10 pillar (Autodesk Fusion 360 design; units mm, degrees)
description: Spur Gear; Module: 1.27; Num Teeth: 11; Pressure Angle: 20.0; Backlash: 0.00 mm
part number: 2026-06-06-15-54-31-604
Autodesk Fusion 360 part; units mm, degrees
pattern_circular "C-Pattern1" [no effect]
sketch "Base Circle" plane through (0, 0, 0) normal (0, 0, 1) x (1, 0, 0)
  circle A0 centre (0, 0) radius 4.8806
  circle A1 centre (0, 0) radius 2.5
extrude "Extrude4" add sketch "Base Circle" along normal blind 1
sketch "Gear Tooth" plane through (0, 0, 0) normal (0, 0, 1) x (1, 0, 0)
  spline S0 degree 5 poles (5.879, -1.0212) (5.8838, -1.022) (5.8935, -1.0235) (5.908, -1.0253) (5.9275, -1.0267) (5.952, -1.0272) (5.9766, -1.0267) (6.0013, -1.0257) (6.026, -1.0244) (6.0508, -1.0228) (6.0756, -1.021) (6.1004, -1.0189) (6.1253, -1.0165) (6.1502, -1.0135) (6.1752, -1.0101) (6.2001, -1.0063) (6.2251, -1.002) (6.2502, -0.9975) (6.2752, -0.9927) (6.3003, -0.9876) (6.3253, -0.9823) (6.3504, -0.9767) (6.3755, -0.9708) (6.4006, -0.9646) (6.4257, -0.9581) (6.4508, -0.9513) (6.4759, -0.9442) (6.501, -0.9369) (6.5261, -0.9293) (6.5512, -0.9215) (6.5763, -0.9134) (6.6014, -0.9051) (6.6265, -0.8965) (6.6516, -0.8877) (6.6767, -0.8786) (6.7018, -0.8693) (6.7268, -0.8598) (6.7519, -0.85) (6.7769, -0.84) (6.8019, -0.8297) (6.8269, -0.8193) (6.8519, -0.8086) (6.8768, -0.7977) (6.9017, -0.7865) (6.9267, -0.7752) (6.9515, -0.7636) (6.9764, -0.7518) (7.0012, -0.7398) (7.0261, -0.7275) (7.0508, -0.7151) (7.0756, -0.7025) (7.1003, -0.6896) (7.125, -0.6765) (7.1497, -0.6632) (7.1743, -0.6498) (7.1989, -0.6361) (7.2235, -0.6222) (7.248, -0.6081) (7.2725, -0.5938) (7.2969, -0.5793) (7.3213, -0.5646) (7.3457, -0.5497) (7.37, -0.5346) (7.3943, -0.5193) (7.4186, -0.5038) (7.4428, -0.4882) (7.4669, -0.4723) (7.491, -0.4562) (7.5151, -0.44) (7.5391, -0.4236) (7.5631, -0.4069) (7.5822, -0.3935) (7.5966, -0.3833) (7.6061, -0.3765) (7.6109, -0.373) knots 0 0 0 0 0 0 0.01428571 0.02857143 0.04285714 0.05714286 0.07142857 0.08571429 0.1 0.11428571 0.12857143 0.14285714 0.15714286 0.17142857 0.18571429 0.2 0.21428571 0.22857143 0.24285714 0.25714286 0.27142857 0.28571429 0.3 0.31428571 0.32857143 0.34285714 0.35714286 0.37142857 0.38571429 0.4 0.41428571 0.42857143 0.44285714 0.45714286 0.47142857 0.48571429 0.5 0.51428571 0.52857143 0.54285714 0.55714286 0.57142857 0.58571429 0.6 0.61428571 0.62857143 0.64285714 0.65714286 0.67142857 0.68571429 0.7 0.71428571 0.72857143 0.74285714 0.75714286 0.77142857 0.78571429 0.8 0.81428571 0.82857143 0.84285714 0.85714286 0.87142857 0.88571429 0.9 0.91428571 0.92857143 0.94285714 0.95714286 0.97142857 0.98571429 1 1 1 1 1 1
  spline S1 degree 5 poles (5.879, 1.0212) (5.8838, 1.022) (5.8935, 1.0235) (5.908, 1.0253) (5.9275, 1.0267) (5.952, 1.0272) (5.9766, 1.0267) (6.0013, 1.0257) (6.026, 1.0244) (6.0508, 1.0228) (6.0756, 1.021) (6.1004, 1.0189) (6.1253, 1.0165) (6.1502, 1.0135) (6.1752, 1.0101) (6.2001, 1.0063) (6.2251, 1.002) (6.2502, 0.9975) (6.2752, 0.9927) (6.3003, 0.9876) (6.3253, 0.9823) (6.3504, 0.9767) (6.3755, 0.9708) (6.4006, 0.9646) (6.4257, 0.9581) (6.4508, 0.9513) (6.4759, 0.9442) (6.501, 0.9369) (6.5261, 0.9293) (6.5512, 0.9215) (6.5763, 0.9134) (6.6014, 0.9051) (6.6265, 0.8965) (6.6516, 0.8877) (6.6767, 0.8786) (6.7018, 0.8693) (6.7268, 0.8598) (6.7519, 0.85) (6.7769, 0.84) (6.8019, 0.8297) (6.8269, 0.8193) (6.8519, 0.8086) (6.8768, 0.7977) (6.9017, 0.7865) (6.9267, 0.7752) (6.9515, 0.7636) (6.9764, 0.7518) (7.0012, 0.7398) (7.0261, 0.7275) (7.0508, 0.7151) (7.0756, 0.7025) (7.1003, 0.6896) (7.125, 0.6765) (7.1497, 0.6632) (7.1743, 0.6498) (7.1989, 0.6361) (7.2235, 0.6222) (7.248, 0.6081) (7.2725, 0.5938) (7.2969, 0.5793) (7.3213, 0.5646) (7.3457, 0.5497) (7.37, 0.5346) (7.3943, 0.5193) (7.4186, 0.5038) (7.4428, 0.4882) (7.4669, 0.4723) (7.491, 0.4562) (7.5151, 0.44) (7.5391, 0.4236) (7.5631, 0.4069) (7.5822, 0.3935) (7.5966, 0.3833) (7.6061, 0.3765) (7.6109, 0.373) knots 0 0 0 0 0 0 0.01428571 0.02857143 0.04285714 0.05714286 0.07142857 0.08571429 0.1 0.11428571 0.12857143 0.14285714 0.15714286 0.17142857 0.18571429 0.2 0.21428571 0.22857143 0.24285714 0.25714286 0.27142857 0.28571429 0.3 0.31428571 0.32857143 0.34285714 0.35714286 0.37142857 0.38571429 0.4 0.41428571 0.42857143 0.44285714 0.45714286 0.47142857 0.48571429 0.5 0.51428571 0.52857143 0.54285714 0.55714286 0.57142857 0.58571429 0.6 0.61428571 0.62857143 0.64285714 0.65714286 0.67142857 0.68571429 0.7 0.71428571 0.72857143 0.74285714 0.75714286 0.77142857 0.78571429 0.8 0.81428571 0.82857143 0.84285714 0.85714286 0.87142857 0.88571429 0.9 0.91428571 0.92857143 0.94285714 0.95714286 0.97142857 0.98571429 1 1 1 1 1 1
  arc A0 (7.6109, -0.373) -> (7.6109, 0.373) centre (0, 0) ccw
  line L0 (4.7988, -0.8335) -> (5.879, -1.0212)
  line L1 (4.7988, 0.8335) -> (5.879, 1.0212)
  line L2 (4.7988, -0.8335) -> (4.7988, 0.8335)
  point P0 (5.998, -1.0258)
  point P1 (6.1192, -1.017)
  point P2 (6.2418, -0.999)
  point P3 (6.3654, -0.9731)
  point P4 (6.4896, -0.9402)
  point P5 (6.6144, -0.9006)
  point P6 (6.7395, -0.8548)
  point P7 (6.8648, -0.8029)
  point P8 (6.9901, -0.7452)
  point P9 (7.1151, -0.6817)
  point P10 (7.2399, -0.6127)
  point P11 (7.3642, -0.5382)
  point P12 (7.4879, -0.4583)
  point P13 (5.998, 1.0258)
  point P14 (6.1192, 1.017)
  point P15 (6.2418, 0.999)
  point P16 (6.3654, 0.9731)
  point P17 (6.4896, 0.9402)
  point P18 (6.6144, 0.9006)
  point P19 (6.7395, 0.8548)
  point P20 (6.8648, 0.8029)
  point P21 (6.9901, 0.7452)
  point P22 (7.1151, 0.6817)
  point P23 (7.2399, 0.6127)
  point P24 (7.3642, 0.5382)
  point P25 (7.4879, 0.4583)
extrude "Extrude5" add sketch "Gear Tooth" along normal blind 1
fillet "Fillet2" radius 0.2 2 edges at (4.8086, -0.8353, 0.5) (4.8086, 0.8353, 0.5)
pattern_circular "C-Pattern2" count 10 over 360 about axis through (0, 0, 0) along (0, 0, 1) of "Extrude5", "Fillet2"
sketch "Diametrial Pitch Circle" plane through (0, 0, 0) normal (0, 0, 1) x (1, 0, 0)
  circle A0 centre (0, 0) radius 6.35 construction
extrude "Extrude6" add 1 faces at (4.0508, 0, 1) along direction (0, 0, 1) blind 17
named bodies: "Spur Gear (10 teeth)"
